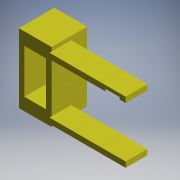
# Autodesk Inventor part: Upper_leg
Saved by Autodesk Inventor 2017 (Build 210142000, 142)
## iProperties
Part Number: Upper_leg
Material: Generic
Document SubType Name: Modeling
Designer: alex-
Appearance: Canary
Author: alex-
Autodesk Inventor part; units mm, degrees
ref_plane "YZ Plane" through (0, 0, 0) normal (1, 0, 0) x (0, 1, 0)
ref_plane "XZ Plane" through (0, 0, 0) normal (0, 1, 0) x (-1, 0, 0)
ref_plane "XY Plane" through (0, 0, 0) normal (0, 0, 1) x (1, 0, 0)
sketch "Sketch1" plane through (0, 0, 0) normal (0, 1, 0) x (-1, 0, 0)
  line L0 (15, 16.25) -> (-15, 16.25)
  line L1 (-15, 16.25) -> (-15, -16.25)
  line L2 (-15, -16.25) -> (15, -16.25)
  line L3 (15, -16.25) -> (15, 16.25)
  point P0 (0, 0)
  point P1 (15, 0)
  point P2 (0, 16.25)
  dimension "d0" = 32.5
  dimension "d1" = 30
  constraints: 8 end point, 2 midpoint, 2 parallel, 1 horizontal, 1 horizontal alignment, 1 perpendicular, 1 vertical alignment
  measures "d0" distance of L2.end L0.start
  measures "d1" distance of L0.end L0.start
extrude "Extrusion1" add sketch "Sketch1" along normal blind 63.5
sketch "Sketch2" plane through (-15, 0, 16.25) normal (0, 0, 1) x (1, 0, 0)
  line L0 (5, 52) -> (25, 52)
  line L1 (25, 52) -> (25, 11.5)
  line L2 (25, 11.5) -> (5, 11.5)
  line L3 (5, 11.5) -> (5, 52)
  line L4 (0, 0) -> (30, 0) projected
  point P0 (15, 0)
  point P1 (15, 11.5)
  point P2 (15, 0)
  dimension "d4" = 40.5
  dimension "d5" = 20
  dimension "d6" = 11.5
  constraints: 8 end point, 2 midpoint, 2 parallel, 1 horizontal, 1 perpendicular, 1 vertical alignment
  measures "d4" distance of L2.end L0.start
  measures "d5" distance of L0.start L0.end
  measures "d6" distance between parallel lines of L4 L2
extrude "Extrusion2" cut sketch "Sketch2" against normal blind 27.5
sketch "Sketch4" plane through (0, 0, 0) normal (0, -1, 0) x (1, 0, 0)
  line L0 (-3.75, -3.25) -> (3.75, -3.25)
  line L1 (3.75, -3.25) -> (3.75, -8.25)
  line L2 (3.75, -8.25) -> (-3.75, -8.25)
  line L3 (-3.75, -8.25) -> (-3.75, -3.25)
  line L4 (15, -16.25) -> (-15, -16.25) projected
  point P0 (0, 0)
  point P1 (0, -3.25)
  dimension "d12" = 5
  dimension "d13" = 7.5
  dimension "d14" = 8
  constraints: 8 end point, 2 parallel, 1 horizontal, 1 midpoint, 1 perpendicular, 1 vertical alignment
  measures "d12" distance of L2.end L0.start
  measures "d13" distance of L0.start L0.end
  measures "d14" distance between parallel lines of L4 L2
extrude "Extrusion4" cut sketch "Sketch4" against normal up to surface (11.5 mm away)
sketch "Sketch5" plane through (15, 0, 16.25) normal (1, 0, 0) x (0, 0, -1)
  line L0 (-2, 60) -> (18, 60)
  line L1 (18, 60) -> (18, 55)
  line L2 (18, 55) -> (-2, 55)
  line L3 (-2, 55) -> (-2, 60)
  line L4 (-2, 8.5) -> (18, 8.5)
  line L5 (18, 8.5) -> (18, 3.5)
  line L6 (18, 3.5) -> (-2, 3.5)
  line L7 (-2, 3.5) -> (-2, 8.5)
  line L8 (32.5, 0) -> (32.5, 63.5) projected
  line L9 (32.5, 0) -> (0, 0) construction
  line L10 (8, 0) -> (8, 63.5) construction
  line L11 (0, 63.5) -> (32.5, 63.5) construction
  line L12 (8, 55) -> (8, 8.5) construction
  point P0 (16.25, 0)
  point P1 (8, 60)
  point P2 (8, 31.75)
  dimension "d17" = 5
  dimension "d18" = 46.5
  dimension "d19" = 20
  dimension "d21" = 24.5
  constraints: 20 end point, 7 point on line, 5 midpoint, 4 parallel, 2 horizontal, 2 perpendicular, 1 collinear, 1 vertical
  measures "d17" distance of L2.end L0.start
  measures "d18" distance of L4.start L2.end
  measures "d19" distance between parallel lines of L1 L3
  measures "d21" distance between parallel lines of L8 L10
extrude "Extrusion5" add sketch "Sketch5" along normal blind 70
sketch "Sketch6" plane through (15, 55, -1.75) normal (0, -1, 0) x (1, 0, 0)
  circle A0 centre (58, 10) radius 12
  line L0 (70, 20) -> (70, 0) projected
  point P0 (-15, 1.75)
  point P1 (70, 10)
  dimension "d24" = 24
  constraints: 1 centre point, 1 horizontal alignment, 1 midpoint, 1 tangent
  measures "d24" diameter of A0
extrude "Extrusion6" cut sketch "Sketch6" against normal blind 2
equation "\"d0\" = b_mat_thickness + s_height - s_land_dist_top - s_land_thickness"
equation "\"d1\" = s_depth + 2 * b_mat_thickness"
equation "\"d2\" = 2 * b_mat_thickness + s_width + 2 * s_land"
equation "\"d4\" = s_width"
equation "\"d5\" = s_depth"
equation "\"d6\" = s_land + b_mat_thickness"
equation "\"d7\" = -s_land_dist_top + s_height - s_land_thickness"
equation "\"d12\" = s_cable_height"
equation "\"d13\" = s_cable_width"
equation "\"d14\" = s_cable_dist_bottom + b_mat_thickness"
equation "\"d17\" = b_mat_thickness"
equation "\"d18\" = s_shaft_height + s_height + 0.5 * b_mat_thickness"
equation "\"d19\" = s_depth"
equation "\"d21\" = 0.5 * b_mat_thickness + 0.5 * s_height + 0.5 * s_shaft_height"
equation "\"d24\" = sa_diameter"
equation "\"d25\" = sa_thickness"
equation "\"b_mat_thickness\" = 5"
equation "\"s_height\" = 38"
equation "\"s_land_dist_top\" = 8"
equation "\"s_land_thickness\" = 2.5"
equation "\"s_depth\" = 20"
equation "\"s_width\" = 40.5"
equation "\"s_land\" = 6.5"
equation "\"s_cable_height\" = 5"
equation "\"s_cable_width\" = 7.5"
equation "\"s_cable_dist_bottom\" = 3"
equation "\"s_shaft_height\" = 6"
equation "\"sa_diameter\" = 24"
equation "\"sa_thickness\" = 2"
body "Solid1"
